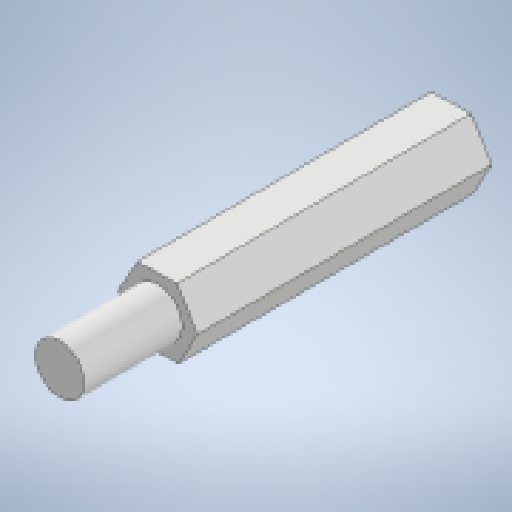
# Autodesk Inventor part: M2_12MM_spacer
Saved by Autodesk Inventor 2024.2 (Build 282272000, 272)
## iProperties
Created: 2024-01-18
Part Number: M2_12MM_spacer
Material: Generic
Document SubType Name: Modeling
Designer: l1534
Density: 1 g/cm^3
Appearance: Default
Author: l1534
Autodesk Inventor part; units mm, degrees
ref_plane "YZ Plane" through (0, 0, 0) normal (1, 0, 0) x (0, 1, 0)
ref_plane "XZ Plane" through (0, 0, 0) normal (0, 1, 0) x (-1, 0, 0)
ref_plane "XY Plane" through (0, 0, 0) normal (0, 0, 1) x (1, 0, 0)
sketch "Sketch1" plane through (0, 0, 0) normal (0, 0, 1) x (1, 0, 0)
  line L0 (-0.8389, 1.3819) -> (0.7773, 1.4175)
  line L1 (0.7773, 1.4175) -> (1.6162, 0.0356)
  line L2 (1.6162, 0.0356) -> (0.8389, -1.3819)
  line L3 (0.8389, -1.3819) -> (-0.7773, -1.4175)
  line L4 (-0.7773, -1.4175) -> (-1.6162, -0.0356)
  line L5 (-1.6162, -0.0356) -> (-0.8389, 1.3819)
  point P0 (0, 0)
  point P1 (0, 0)
  dimension "d0" = 1.4
  constraints: 12 end point, 1 coincident, 13 other
  measures "d0" distance from line of L0 point (0, 0)
extrude "Extrusion1" add sketch "Sketch1" along normal blind 12
sketch "Sketch2" plane through (0, 0, 12) normal (0, 0, 1) x (1, 0, 0)
  circle A0 centre (0, 0) radius 1
  dimension "d3" = 2
  constraints: 1 centre point, 1 coincident
  measures "d3" diameter of A0
extrude "Extrusion2" add sketch "Sketch2" along normal blind 4
body "Solid1"
